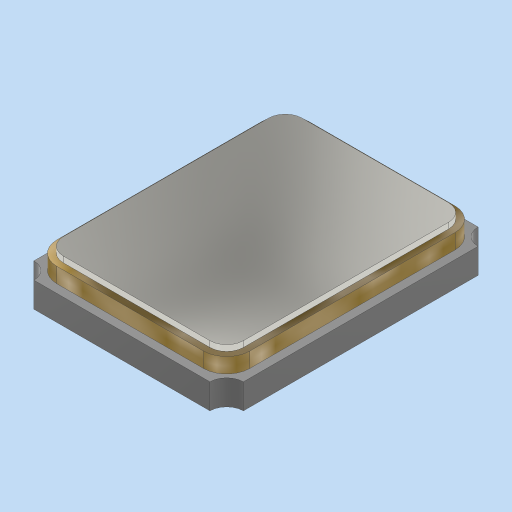
# Autodesk Inventor part: crystal_oscillator
Saved by Autodesk Inventor 2024 (Build 280153000, 153)
## iProperties
Created: 2025-05-06
Part Number: crystal_oscillator
Material: Generic
Document SubType Name: Modeling
Designer: XxPan
Density: 1 g/cm^3
Appearance: Default
Author: XxPan
Autodesk Inventor part; units mm, degrees
ref_plane "YZ Plane" through (0, 0, 0) normal (1, 0, 0) x (0, 1, 0)
ref_plane "XZ Plane" through (0, 0, 0) normal (0, 1, 0) x (-1, 0, 0)
ref_plane "XY Plane" through (0, 0, 0) normal (0, 0, 1) x (1, 0, 0)
sketch "Sketch1" plane through (0, 0, 0) normal (0, 1, 0) x (-1, 0, 0)
  line L0 (1.25, 1.6) -> (-1.25, 1.6)
  line L1 (-1.25, 1.6) -> (-1.25, -1.6)
  line L2 (-1.25, -1.6) -> (1.25, -1.6)
  line L3 (1.25, -1.6) -> (1.25, 1.6)
  line L4 (1.75, 0) -> (-1.75, 0) construction
  line L5 (0, -2.24) -> (0, 2.24) construction
  point P0 (0, 0)
  dimension "d0" = 3.2
  dimension "d1" = 2.5
  constraints: 8 end point, 2 parallel, 1 horizontal, 1 perpendicular, 2 other
  measures "d0" distance of L2.end L0.start
  measures "d1" distance of L0.start L0.end
extrude "Extrusion1" add sketch "Sketch1" along normal blind 0.3
sketch "Sketch2" plane through (0, 0.3, 0) normal (0, 1, 0) x (1, 0, 0)
  line L0 (-1.15, -1.5) -> (1.15, -1.5)
  line L1 (1.15, -1.5) -> (1.15, 1.5)
  line L2 (1.15, 1.5) -> (-1.15, 1.5)
  line L3 (-1.15, 1.5) -> (-1.15, -1.5)
  line L4 (-1.75, 0) -> (1.75, 0) construction
  line L5 (0, 2.24) -> (0, -2.24) construction
  point P0 (0, 0)
  dimension "d4" = 2.3
  dimension "d5" = 3
  constraints: 8 end point, 2 parallel, 1 horizontal, 1 perpendicular, 2 other
  measures "d4" distance of L2.end L1.end
  measures "d5" distance of L1.end L0.end
extrude "Extrusion2" add sketch "Sketch2" along normal blind 0.18
sketch "Sketch3" plane through (0, 0.48, 0) normal (0, 1, 0) x (1, 0, 0)
  line L0 (-1.075, -1.425) -> (1.075, -1.425)
  line L1 (1.075, -1.425) -> (1.075, 1.425)
  line L2 (1.075, 1.425) -> (-1.075, 1.425)
  line L3 (-1.075, 1.425) -> (-1.075, -1.425)
  line L4 (-1.75, 0) -> (1.75, 0) construction
  line L5 (0, 2.24) -> (0, -2.24) construction
  point P0 (0, 0)
  dimension "d8" = 2.85
  dimension "d9" = 2.15
  constraints: 8 end point, 2 parallel, 1 horizontal, 1 perpendicular, 2 other
  measures "d8" distance of L2.end L0.start
  measures "d9" distance of L1.end L2.end
extrude "Extrusion3" add sketch "Sketch3" along normal blind 0.07
fillet "Fillet1" radius 0.2 4 edges at (1.075, 0.515, 1.425) (1.075, 0.515, -1.425) (-1.075, 0.515, -1.425) (-1.075, 0.515, 1.425)
fillet "Fillet2" radius 0.275 4 edges at (1.15, 0.39, 1.5) (1.15, 0.39, -1.5) (-1.15, 0.39, -1.5) (-1.15, 0.39, 1.5)
fillet "Fillet3" radius 0.2 4 edges at (1.25, 0.15, 1.6) (1.25, 0.15, -1.6) (-1.25, 0.15, -1.6) (-1.25, 0.15, 1.6) inverted yes
body "Solid1"
